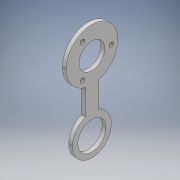
# Autodesk Inventor part: barrecodeuse
Saved by Autodesk Inventor 2017 SP1 (Build 210196100, 196)
## iProperties
Part Number: barrecodeuse
Material: Générique
Document SubType Name: Modeling
Designer: Sylvain
Density: 1 g/cm^3
Appearance: Par défaut
Author: Sylvain
## iProperties of the stored document barrecodeuse_Impression 3D.ipt
Part Number: barrecodeuse_Impression 3D
Material: Générique
Document SubType Name: Modeling
Designer: Sylvain
Density: 1 g/cm^3
Appearance: Par défaut
Author: Sylvain
Autodesk Inventor part; units mm, degrees
ref_plane "YZ Plane" through (0, 0, 0) normal (1, 0, 0) x (0, 1, 0)
ref_plane "XZ Plane" through (0, 0, 0) normal (0, 1, 0) x (-1, 0, 0)
ref_plane "XY Plane" through (0, 0, 0) normal (0, 0, 1) x (1, 0, 0)
sketch "Esquisse1" plane through (0, 0, 0) normal (1, 0, 0) x (0, 1, 0)
  line L0 (0, 0) -> (10, 0)
  line L1 (10, 0) -> (10, -65)
  line L2 (10, -65) -> (0, -65)
  line L3 (0, -65) -> (0, 0)
  point P0 (5, -5)
  point P1 (5, -54.2442)
  dimension "d0" = 65
  dimension "d1" = 10
  dimension "d2" = 5
  dimension "d3" = 5
  dimension "d4" = 49.2442
  dimension "d5" = 5
  constraints: 8 end point, 2 parallel, 1 horizontal, 1 perpendicular
  measures "d0" distance of L2.end L0.start
  measures "d1" distance of L1.end L2.end
  measures "d2" distance from line of L0 point (5, -5)
  measures "d3" distance from line of L3 point (5, -5)
  measures "d4" distance of point (5, -54.244) point (5, -5)
  measures "d5" distance from line of L3 point (5, -54.244)
extrude "Extrusion1" add sketch "Esquisse1" along normal blind 3
sketch "Esquisse2" plane through (0, 0, 0) normal (-1, 0, 0) x (0, 0, 1)
  line L0 (-25, 25) -> (15, 25)
  line L1 (15, 25) -> (15, -15)
  line L2 (15, -15) -> (-25, -15)
  line L3 (-25, -15) -> (-25, 25)
  line L4 (-65, 0) -> (0, 0) projected
  line L5 (0, 0) -> (0, 10) projected
  line L6 (-50, -10) -> (-80, -10)
  line L7 (-80, -10) -> (-80, 20)
  line L8 (-80, 20) -> (-50, 20)
  line L9 (-50, 20) -> (-50, -10)
  line L10 (-65, 10) -> (-65, 0) projected
  dimension "d8" = 40
  dimension "d9" = 25
  dimension "d10" = 40
  dimension "d11" = 25
  dimension "d36" = 30
  dimension "d37" = 30
  dimension "d38" = 20
  dimension "d39" = 15
  constraints: 16 end point, 4 parallel, 2 horizontal, 2 perpendicular
  measures "d8" distance of L2.end L0.start
  measures "d9" distance between parallel lines of L4 L0
  measures "d10" distance of L0.start L0.end
  measures "d11" distance between parallel lines of L5 L3
  measures "d36" distance of L7.end L8.end
  measures "d37" distance of L6.end L7.end
  measures "d38" distance between parallel lines of L4 L8
  measures "d39" distance between parallel lines of L10 L7
extrude "Extrusion2" add sketch "Esquisse2" against normal blind 3 contours L0 L1 L2 L3
sketch "Esquisse3" plane through (0, 0, 0) normal (-1, 0, 0) x (0, 0, 1)
  line L0 (-65, 10) -> (-25, 10) projected
  line L1 (-65, 10) -> (-65, 0) projected
  line L2 (-65, 0) -> (-25, 0) projected
  circle A0 centre (-60, 5) radius 4
  circle A1 centre (-6.1484, 5) radius 10
  point P0 (0, 0)
  dimension "d14" = 5
  dimension "d15" = 5
  dimension "d16" = 53.8516
  dimension "d17" = 5
  dimension "d18" = 8
  dimension "d19" = 20
  constraints: 2 centre point, 2 coincident
  measures "d14" distance from line of L0 point (-60, 5)
  measures "d15" distance from line of L1 point (-60, 5)
  measures "d16" distance of point (-6.148, 5) point (-60, 5)
  measures "d17" distance from line of L2 point (-6.148, 5)
  measures "d18" diameter of A0
  measures "d19" diameter of A1
extrude "Extrusion3" cut sketch "Esquisse3" against normal blind 3
sketch "Esquisse4" plane through (0, 0, 0) normal (-1, 0, 0) x (0, 0, 1)
  circle A0 centre (-6.1484, 5) radius 10 projected
  circle A1 centre (-6.1484, 5) radius 15
  point P0 (0, 0)
  point P1 (-6.1484, 20)
  point P2 (-19.1388, -2.5)
  point P3 (6.842, -2.5)
  dimension "d22" = 30
  dimension "d25" = 360
  constraints: 1 coincident, 1 vertical alignment, 6 other
hole "Perçage1" at (0, 20, -6.1484) at (0, -2.5, -19.1388) at (0, -2.5, 6.842) direction (1, 0, 0) diameter 3.5 depth 3 tip angle 118
fillet "Congé1" radius 3 2 edges at (1.5, 10, -65) (1.5, 0, -65)
fillet "Congé2" radius 20 4 edges at (1.5, -15, -25) (1.5, 25, -25) (1.5, -15, 15) (1.5, 25, 15)
sketch "Esquisse5" plane through (0, 0, 0) normal (-1, 0, 0) x (0, 0, 1)
  line L0 (-75, 20) -> (-45, 20)
  line L1 (-45, 20) -> (-45, -10)
  line L2 (-45, -10) -> (-75, -10)
  line L3 (-75, -10) -> (-75, 20)
  line L4 (-62, 0) -> (-25, 0) projected
  line L5 (-65, 7) -> (-65, 3) projected
  point P0 (0, 0)
  dimension "d40" = 30
  dimension "d41" = 30
  dimension "d42" = 20
  dimension "d43" = 10
  constraints: 8 end point, 2 parallel, 1 horizontal, 1 perpendicular
  measures "d40" distance of L0.start L0.end
  measures "d41" distance of L2.end L0.start
  measures "d42" distance between parallel lines of L4 L0
  measures "d43" distance between parallel lines of L5 L3
extrude "Extrusion4" add sketch "Esquisse5" against normal blind 3
sketch "Esquisse6" plane through (0, 0, 0) normal (-1, 0, 0) x (0, 0, 1)
  line L0 (-75, 20) -> (-45, 20) projected
  circle A0 centre (-6.1484, 5) radius 10 projected
  point P0 (0, 0)
  point P1 (-60, 5)
  dimension "d46" = 15
  dimension "d47" = 53.8516
  measures "d46" distance from line of L0 point (-60, 5)
  measures "d47" distance of A0.centre point (-60, 5)
hole "Perçage2" at (0, 5, -60) direction (1, 0, 0) diameter 22 depth 3 tip angle 118
fillet "Congé3" radius 15 4 edges at (1.5, -10, -75) (1.5, -10, -45) (1.5, 20, -45) (1.5, 20, -75)
